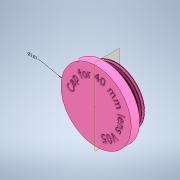
# Autodesk Inventor part: capForSvBonyPlosse-40mmV05
Saved by Autodesk Inventor 2021.1 (Build 251245010, 245A)
## iProperties
Created: 2020-08-18
Part Number: capForSvBonyPlosse-40mmV05
Material: Polycarbonate, Smoke
Document SubType Name: Modeling
Designer: robst
Density: 1.2 g/cm^3
Appearance: Pink
innerDiameter: 0.635 in
heightOfBrake: 0.250 in
majorDiameter: 1.623 in
pitchDiameter: 1.569 in
minorDiameter: 1.524 in
pitch: 0.083 in
crestFlat: 0.017 in
threadsPerInch: 12.000 ul
threadDepth: 0.060 in
Author: robst
Autodesk Inventor part; units mm, degrees
ref_plane "XZ Plane" through (0, 0, 0) normal (0, 1, 0) x (-1, 0, 0)
ref_plane "XY Plane" through (0, 0, 0) normal (0, 0, 1) x (1, 0, 0)
sketch "Sketch1" plane through (0, 0, 0) normal (0, 0, 1) x (1, 0, 0)
  circle A0 centre (0, 0) radius 21.2992
  dimension "d1" = 42.5983
  constraints: 1 centre point
  measures "d1" diameter of A0
extrude "Extrusion1" add sketch "Sketch1" against normal blind 9.525
sketch "Sketch2" plane through (0, 0, 0) normal (0, 0, 1) x (1, 0, 0)
  circle A0 centre (0, 0) radius 26.3436
  dimension "d4" = 52.6872
  constraints: 1 centre point
  measures "d4" diameter of A0
extrude "Extrusion2" add sketch "Sketch2" along normal blind 6.35
sketch "Sketch11" plane through (0, 0, 6.35) normal (0, 0, 1) x (1, 0, 0)
  circle A0 centre (0, 0) radius 19.05 construction
  spline S0 degree 2 poles (-16.2379, 2.4675) (-16.3002, 1.9774) (-16.7363, 1.1904) (-17.1055, 0.9302) knots 0 0 0 1 2 2 2
  spline S1 degree 2 poles (-17.1055, 0.9302) (-17.4706, 0.6695) (-18.4927, 0.4633) (-19.1298, 0.5442) knots 0 0 0 1 2 2 2
  spline S2 degree 2 poles (-19.1298, 0.5442) (-19.7628, 0.6246) (-20.6611, 1.0666) (-20.9693, 1.417) knots 0 0 0 1 2 2 2
  spline S3 degree 2 poles (-20.9693, 1.417) (-21.2699, 1.7622) (-21.5204, 2.6323) (-21.4556, 3.1428) knots 0 0 0 1 2 2 2
  spline S4 degree 2 poles (-21.4556, 3.1428) (-21.4234, 3.396) (-21.2933, 3.8318) (-21.2123, 4.0124) knots 0 0 0 1 2 2 2
  spline S5 degree 2 poles (-21.2123, 4.0124) (-21.1384, 4.169) (-20.9443, 4.4888) (-20.8332, 4.6448) knots 0 0 0 1 2 2 2
  line L0 (-20.8332, 4.6448) -> (-20.0246, 4.5421)
  line L1 (-20.0246, 4.5421) -> (-20.0313, 4.489)
  spline S6 degree 2 poles (-20.0313, 4.489) (-20.1244, 4.4095) (-20.3884, 4.1609) (-20.5241, 3.9748) knots 0 0 0 1 2 2 2
  spline S7 degree 2 poles (-20.5241, 3.9748) (-20.6546, 3.7963) (-20.847, 3.3601) (-20.8843, 3.0661) knots 0 0 0 1 2 2 2
  spline S8 degree 2 poles (-20.8843, 3.0661) (-20.9253, 2.7435) (-20.733, 2.1339) (-20.5073, 1.8853) knots 0 0 0 1 2 2 2
  spline S9 degree 2 poles (-20.5073, 1.8853) (-20.277, 1.6402) (-19.5271, 1.3043) (-19.0411, 1.2425) knots 0 0 0 1 2 2 2
  spline S10 degree 2 poles (-19.0411, 1.2425) (-18.5225, 1.1767) (-17.7435, 1.3308) (-17.4587, 1.5146) knots 0 0 0 1 2 2 2
  spline S11 degree 2 poles (-17.4587, 1.5146) (-17.1826, 1.6953) (-16.8573, 2.2308) (-16.8168, 2.5493) knots 0 0 0 1 2 2 2
  spline S12 degree 2 poles (-16.8168, 2.5493) (-16.78, 2.8393) (-16.8601, 3.3516) (-16.9419, 3.557) knots 0 0 0 1 2 2 2
  spline S13 degree 2 poles (-16.9419, 3.557) (-17.0248, 3.7543) (-17.2105, 4.0559) (-17.2783, 4.1434) knots 0 0 0 1 2 2 2
  line L2 (-17.2783, 4.1434) -> (-17.272, 4.1924)
  line L3 (-17.272, 4.1924) -> (-16.4716, 4.0907)
  spline S14 degree 2 poles (-16.4716, 4.0907) (-16.4153, 3.9134) (-16.3097, 3.6012) (-16.2708, 3.3846) knots 0 0 0 1 2 2 2
  spline S15 degree 2 poles (-16.2708, 3.3846) (-16.2253, 3.1548) (-16.1995, 2.7697) (-16.2379, 2.4675) knots 0 0 0 1 2 2 2
  spline S16 degree 2 poles (-15.5406, 6.7174) (-15.5146, 6.6238) (-15.4158, 6.3044) (-15.402, 6.167) knots 0 0 0 1 2 2 2
  spline S17 degree 2 poles (-15.402, 6.167) (-15.3773, 5.977) (-15.4015, 5.6471) (-15.5039, 5.3777) knots 0 0 0 1 2 2 2
  spline S18 degree 2 poles (-15.5039, 5.3777) (-15.5873, 5.1584) (-15.9035, 4.825) (-16.1106, 4.732) knots 0 0 0 1 2 2 2
  spline S19 degree 2 poles (-16.1106, 4.732) (-16.311, 4.6452) (-16.8078, 4.6359) (-17.0463, 4.7266) knots 0 0 0 1 2 2 2
  spline S20 degree 2 poles (-17.0463, 4.7266) (-17.4157, 4.8671) (-17.8205, 5.3778) (-17.8418, 5.7735) knots 0 0 0 1 2 2 2
  spline S21 degree 2 poles (-17.8418, 5.7735) (-17.8662, 6.1263) (-17.66, 6.9815) (-17.5069, 7.4651) knots 0 0 0 1 2 2 2
  line L4 (-17.5069, 7.4651) -> (-17.6224, 7.509)
  spline S22 degree 2 poles (-17.6224, 7.509) (-17.8301, 7.588) (-18.1362, 7.559) (-18.2532, 7.4714) knots 0 0 0 1 2 2 2
  spline S23 degree 2 poles (-18.2532, 7.4714) (-18.3702, 7.3837) (-18.5423, 7.0704) (-18.6096, 6.8934) knots 0 0 0 1 2 2 2
  spline S24 degree 2 poles (-18.6096, 6.8934) (-18.6886, 6.6856) (-18.7791, 6.077) (-18.7666, 5.7507) knots 0 0 0 1 2 2 2
  line L5 (-18.7666, 5.7507) -> (-18.7797, 5.7161)
  line L6 (-18.7797, 5.7161) -> (-19.3916, 5.9487)
  spline S25 degree 2 poles (-19.3916, 5.9487) (-19.3748, 6.1317) (-19.2547, 6.7951) (-19.1391, 7.0991) knots 0 0 0 1 2 2 2
  spline S26 degree 2 poles (-19.1391, 7.0991) (-18.9986, 7.4685) (-18.6915, 7.9287) (-18.4654, 8.0717) knots 0 0 0 1 2 2 2
  spline S27 degree 2 poles (-18.4654, 8.0717) (-18.2445, 8.2124) (-17.7058, 8.2277) (-17.371, 8.1004) knots 0 0 0 1 2 2 2
  line L7 (-17.371, 8.1004) -> (-14.9353, 7.1743)
  line L8 (-14.9353, 7.1743) -> (-15.1635, 6.574)
  line L9 (-15.1635, 6.574) -> (-15.5406, 6.7174)
  line L10 (-16.0409, 6.9076) -> (-17.0298, 7.2836)
  spline S28 degree 2 poles (-17.0298, 7.2836) (-17.0925, 7.0608) (-17.2743, 6.3857) (-17.2903, 6.1583) knots 0 0 0 1 2 2 2
  spline S29 degree 2 poles (-17.2903, 6.1583) (-17.3079, 5.8919) (-17.1224, 5.4647) (-16.8531, 5.3623) knots 0 0 0 1 2 2 2
  spline S30 degree 2 poles (-16.8531, 5.3623) (-16.5453, 5.2452) (-16.1019, 5.473) (-15.9761, 5.8039) knots 0 0 0 1 2 2 2
  spline S31 degree 2 poles (-15.9761, 5.8039) (-15.8693, 6.0848) (-15.9361, 6.6387) (-16.0409, 6.9076) knots 0 0 0 1 2 2 2
  spline S32 degree 2 poles (-14.4215, 11.7457) (-13.6281, 11.2141) (-13.1975, 9.8303) (-13.5848, 9.2524) knots 0 0 0 1 2 2 2
  spline S33 degree 2 poles (-13.5848, 9.2524) (-13.7429, 9.0164) (-14.0953, 8.7273) (-14.3342, 8.6148) knots 0 0 0 1 2 2 2
  line L11 (-14.3342, 8.6148) -> (-13.0073, 7.7256)
  line L12 (-13.0073, 7.7256) -> (-13.3648, 7.1921)
  line L13 (-13.3648, 7.1921) -> (-17.6977, 10.0958)
  line L14 (-17.6977, 10.0958) -> (-17.3402, 10.6292)
  line L15 (-17.3402, 10.6292) -> (-17.0085, 10.4069)
  spline S34 degree 2 poles (-17.0085, 10.4069) (-17.0568, 10.7268) (-16.9708, 11.3728) (-16.7806, 11.6566) knots 0 0 0 1 2 2 2
  spline S35 degree 2 poles (-16.7806, 11.6566) (-16.4162, 12.2004) (-15.1465, 12.2316) (-14.4215, 11.7457) knots 0 0 0 1 2 2 2
  spline S36 degree 2 poles (-14.7289, 11.1539) (-15.2726, 11.5183) (-16.1026, 11.5739) (-16.3615, 11.1875) knots 0 0 0 1 2 2 2
  spline S37 degree 2 poles (-16.3615, 11.1875) (-16.5128, 10.9618) (-16.5952, 10.4025) (-16.5639, 10.109) knots 0 0 0 1 2 2 2
  line L16 (-16.5639, 10.109) -> (-14.7651, 8.9036)
  spline S38 degree 2 poles (-14.7651, 8.9036) (-14.5261, 9.0457) (-14.2515, 9.2928) (-14.1232, 9.4843) knots 0 0 0 1 2 2 2
  spline S39 degree 2 poles (-14.1232, 9.4843) (-13.8459, 9.8981) (-14.1475, 10.7643) (-14.7289, 11.1539) knots 0 0 0 1 2 2 2
  line L17 (-11.9885, 17.5305) -> (-12.0145, 17.5103)
  spline S40 degree 2 poles (-12.0145, 17.5103) (-12.103, 17.4833) (-12.392, 17.3319) (-12.4927, 17.2536) knots 0 0 0 1 2 2 2
  spline S41 degree 2 poles (-12.4927, 17.2536) (-12.8114, 17.0061) (-12.8623, 16.5079) (-12.5694, 16.1308) knots 0 0 0 1 2 2 2
  line L18 (-12.5694, 16.1308) -> (-12.4911, 16.03)
  line L19 (-12.4911, 16.03) -> (-11.6522, 16.6814)
  line L20 (-11.6522, 16.6814) -> (-11.3265, 16.262)
  line L21 (-11.3265, 16.262) -> (-12.1491, 15.6232)
  line L22 (-12.1491, 15.6232) -> (-10.1366, 13.0319)
  line L23 (-10.1366, 13.0319) -> (-10.6438, 12.638)
  line L24 (-10.6438, 12.638) -> (-12.6563, 15.2293)
  line L25 (-12.6563, 15.2293) -> (-12.9977, 14.9641)
  line L26 (-12.9977, 14.9641) -> (-13.3234, 15.3835)
  line L27 (-13.3234, 15.3835) -> (-12.982, 15.6487)
  line L28 (-12.982, 15.6487) -> (-13.0603, 15.7495)
  spline S42 degree 2 poles (-13.0603, 15.7495) (-13.4795, 16.2892) (-13.3954, 17.2615) (-12.9077, 17.6402) knots 0 0 0 1 2 2 2
  spline S43 degree 2 poles (-12.9077, 17.6402) (-12.7679, 17.7488) (-12.4753, 17.9291) (-12.3496, 17.9955) knots 0 0 0 1 2 2 2
  line L29 (-12.3496, 17.9955) -> (-11.9885, 17.5305)
  spline S44 degree 2 poles (-6.8969, 17.1605) (-6.4569, 16.3035) (-6.8014, 14.9466) (-7.4899, 14.5931) knots 0 0 0 1 2 2 2
  spline S45 degree 2 poles (-7.4899, 14.5931) (-8.1967, 14.2302) (-9.5006, 14.7778) (-9.9255, 15.6055) knots 0 0 0 1 2 2 2
  spline S46 degree 2 poles (-9.9255, 15.6055) (-10.3617, 16.4551) (-10.01, 17.825) (-9.3288, 18.1748) knots 0 0 0 1 2 2 2
  spline S47 degree 2 poles (-9.3288, 18.1748) (-8.6403, 18.5282) (-7.3349, 18.0138) (-6.8969, 17.1605) knots 0 0 0 1 2 2 2
  spline S48 degree 2 poles (-7.4865, 16.8577) (-7.8249, 17.5169) (-8.6337, 17.9115) (-9.0768, 17.684) knots 0 0 0 1 2 2 2
  spline S49 degree 2 poles (-9.0768, 17.684) (-9.52, 17.4565) (-9.6743, 16.5674) (-9.3359, 15.9082) knots 0 0 0 1 2 2 2
  spline S50 degree 2 poles (-9.3359, 15.9082) (-9.0069, 15.2673) (-8.185, 14.8563) (-7.7419, 15.0838) knots 0 0 0 1 2 2 2
  spline S51 degree 2 poles (-7.7419, 15.0838) (-7.3024, 15.3095) (-7.1518, 16.2059) (-7.4865, 16.8577) knots 0 0 0 1 2 2 2
  line L30 (-4.3209, 19.1925) -> (-4.3525, 19.1833)
  spline S52 degree 2 poles (-4.3525, 19.1833) (-4.4294, 19.1823) (-4.5859, 19.1452) (-4.6926, 19.1141) knots 0 0 0 1 2 2 2
  spline S53 degree 2 poles (-4.6926, 19.1141) (-4.9415, 19.0414) (-5.3682, 18.6811) (-5.5272, 18.4032) knots 0 0 0 1 2 2 2
  line L31 (-5.5272, 18.4032) -> (-4.7698, 15.8067)
  line L32 (-4.7698, 15.8067) -> (-5.3863, 15.6269)
  line L33 (-5.3863, 15.6269) -> (-6.4539, 19.2864)
  line L34 (-6.4539, 19.2864) -> (-5.8373, 19.4662)
  line L35 (-5.8373, 19.4662) -> (-5.6783, 18.9209)
  spline S54 degree 2 poles (-5.6783, 18.9209) (-5.43, 19.3192) (-4.9995, 19.7107) (-4.7624, 19.7798) knots 0 0 0 1 2 2 2
  spline S55 degree 2 poles (-4.7624, 19.7798) (-4.6676, 19.8075) (-4.5704, 19.8273) (-4.5077, 19.8327) knots 0 0 0 1 2 2 2
  line L36 (-4.5077, 19.8327) -> (-4.3209, 19.1925)
  line L37 (2.4474, 18.1735) -> (1.8427, 18.1972)
  line L38 (1.8427, 18.1972) -> (1.7743, 16.4531)
  line L39 (1.7743, 16.4531) -> (1.1202, 16.4788)
  line L40 (1.1202, 16.4788) -> (1.1886, 18.2229)
  line L41 (1.1886, 18.2229) -> (-1.0532, 18.3108)
  line L42 (-1.0532, 18.3108) -> (-1.0251, 19.0266)
  line L43 (-1.0251, 19.0266) -> (1.3482, 21.5537)
  line L44 (1.3482, 21.5537) -> (1.9734, 21.5292)
  line L45 (1.9734, 21.5292) -> (1.8642, 18.7443)
  line L46 (1.8642, 18.7443) -> (2.4689, 18.7206)
  line L47 (2.4689, 18.7206) -> (2.4474, 18.1735)
  line L48 (1.2101, 18.77) -> (1.2879, 20.7527)
  line L49 (1.2879, 20.7527) -> (-0.497, 18.837)
  line L50 (-0.497, 18.837) -> (1.2101, 18.77)
  spline S56 degree 2 poles (6.632, 17.9322) (6.2687, 16.6146) (5.1624, 15.5916) (4.3647, 15.8116) knots 0 0 0 1 2 2 2
  spline S57 degree 2 poles (4.3647, 15.8116) (3.5551, 16.0349) (3.144, 17.5019) (3.4997, 18.7917) knots 0 0 0 1 2 2 2
  spline S58 degree 2 poles (3.4997, 18.7917) (3.8653, 20.1172) (4.9694, 21.1323) (5.771, 20.9112) knots 0 0 0 1 2 2 2
  spline S59 degree 2 poles (5.771, 20.9112) (6.5766, 20.689) (6.9844, 19.2101) (6.632, 17.9322) knots 0 0 0 1 2 2 2
  spline S60 degree 2 poles (5.3792, 16.672) (5.5412, 16.8878) (5.8263, 17.612) (5.9653, 18.116) knots 0 0 0 1 2 2 2
  spline S61 degree 2 poles (5.9653, 18.116) (6.1043, 18.62) (6.2296, 19.3841) (6.1993, 19.6614) knots 0 0 0 1 2 2 2
  spline S62 degree 2 poles (6.1993, 19.6614) (6.169, 19.9388) (5.8949, 20.292) (5.6211, 20.3675) knots 0 0 0 1 2 2 2
  spline S63 degree 2 poles (5.6211, 20.3675) (5.3473, 20.443) (4.9229, 20.2825) (4.7486, 20.053) knots 0 0 0 1 2 2 2
  spline S64 degree 2 poles (4.7486, 20.053) (4.5804, 19.8303) (4.2989, 19.088) (4.1664, 18.6078) knots 0 0 0 1 2 2 2
  spline S65 degree 2 poles (4.1664, 18.6078) (4.0242, 18.0919) (3.8972, 17.3839) (3.926, 17.0856) knots 0 0 0 1 2 2 2
  spline S66 degree 2 poles (3.926, 17.0856) (3.9512, 16.8053) (4.2289, 16.4341) (4.5146, 16.3553) knots 0 0 0 1 2 2 2
  spline S67 degree 2 poles (4.5146, 16.3553) (4.7845, 16.2809) (5.2088, 16.4414) (5.3792, 16.672) knots 0 0 0 1 2 2 2
  line L51 (11.9604, 11.5312) -> (13.3681, 13.2304)
  spline S68 degree 2 poles (13.3681, 13.2304) (13.5361, 13.4333) (13.7907, 13.8051) (13.8187, 13.9422) knots 0 0 0 1 2 2 2
  spline S69 degree 2 poles (13.8187, 13.9422) (13.8547, 14.0889) (13.7453, 14.3505) (13.5773, 14.4897) knots 0 0 0 1 2 2 2
  spline S70 degree 2 poles (13.5773, 14.4897) (13.4251, 14.6158) (12.9215, 14.7176) (12.5905, 14.6924) knots 0 0 0 1 2 2 2
  spline S71 degree 2 poles (12.5905, 14.6924) (12.5569, 14.6454) (12.4609, 14.5165) (12.3926, 14.4341) knots 0 0 0 1 2 2 2
  line L52 (12.3926, 14.4341) -> (10.7906, 12.5002)
  line L53 (10.7906, 12.5002) -> (10.2961, 12.9099)
  line L54 (10.2961, 12.9099) -> (11.7037, 14.6091)
  spline S72 degree 2 poles (11.7037, 14.6091) (11.8718, 14.812) (12.1263, 15.1839) (12.1544, 15.321) knots 0 0 0 1 2 2 2
  spline S73 degree 2 poles (12.1544, 15.321) (12.1903, 15.4676) (12.081, 15.7293) (11.9129, 15.8684) knots 0 0 0 1 2 2 2
  spline S74 degree 2 poles (11.9129, 15.8684) (11.7544, 15.9998) (11.2371, 16.0915) (10.9435, 16.0728) knots 0 0 0 1 2 2 2
  line L55 (10.9435, 16.0728) -> (9.1262, 13.8789)
  line L56 (9.1262, 13.8789) -> (8.6317, 14.2886)
  line L57 (8.6317, 14.2886) -> (11.0635, 17.2243)
  line L58 (11.0635, 17.2243) -> (11.5581, 16.8146)
  line L59 (11.5581, 16.8146) -> (11.2902, 16.4912)
  spline S75 degree 2 poles (11.2902, 16.4912) (11.6438, 16.5244) (12.2002, 16.4217) (12.4284, 16.2326) knots 0 0 0 1 2 2 2
  spline S76 degree 2 poles (12.4284, 16.2326) (12.6884, 16.0173) (12.894, 15.446) (12.7754, 15.0898) knots 0 0 0 1 2 2 2
  spline S77 degree 2 poles (12.7754, 15.0898) (13.208, 15.1538) (13.8455, 15.0587) (14.0928, 14.8539) knots 0 0 0 1 2 2 2
  spline S78 degree 2 poles (14.0928, 14.8539) (14.283, 14.6963) (14.4965, 14.3216) (14.5004, 14.0939) knots 0 0 0 1 2 2 2
  spline S79 degree 2 poles (14.5004, 14.0939) (14.5074, 13.8636) (14.3064, 13.3565) (14.057, 13.0553) knots 0 0 0 1 2 2 2
  line L60 (14.057, 13.0553) -> (12.455, 11.1215)
  line L61 (12.455, 11.1215) -> (11.9604, 11.5312)
  line L62 (15.2004, 6.7058) -> (17.1072, 7.8162)
  spline S80 degree 2 poles (17.1072, 7.8162) (17.3348, 7.9488) (17.7019, 8.2102) (17.7755, 8.3293) knots 0 0 0 1 2 2 2
  spline S81 degree 2 poles (17.7755, 8.3293) (17.8597, 8.4545) (17.8472, 8.7378) (17.7374, 8.9264) knots 0 0 0 1 2 2 2
  spline S82 degree 2 poles (17.7374, 8.9264) (17.6379, 9.0971) (17.2002, 9.3662) (16.8808, 9.4565) knots 0 0 0 1 2 2 2
  spline S83 degree 2 poles (16.8808, 9.4565) (16.8331, 9.424) (16.6985, 9.3361) (16.606, 9.2822) knots 0 0 0 1 2 2 2
  line L63 (16.606, 9.2822) -> (14.4359, 8.0185)
  line L64 (14.4359, 8.0185) -> (14.1128, 8.5735)
  line L65 (14.1128, 8.5735) -> (16.0195, 9.6839)
  spline S84 degree 2 poles (16.0195, 9.6839) (16.2472, 9.8165) (16.6143, 10.0778) (16.6878, 10.1969) knots 0 0 0 1 2 2 2
  spline S85 degree 2 poles (16.6878, 10.1969) (16.7721, 10.3222) (16.7596, 10.6055) (16.6498, 10.794) knots 0 0 0 1 2 2 2
  spline S86 degree 2 poles (16.6498, 10.794) (16.5462, 10.9719) (16.0921, 11.2363) (15.8101, 11.3197) knots 0 0 0 1 2 2 2
  line L66 (15.8101, 11.3197) -> (13.3483, 9.8862)
  line L67 (13.3483, 9.8862) -> (13.0251, 10.4411)
  line L68 (13.0251, 10.4411) -> (16.3193, 12.3595)
  line L69 (16.3193, 12.3595) -> (16.6425, 11.8045)
  line L70 (16.6425, 11.8045) -> (16.2796, 11.5932)
  spline S87 degree 2 poles (16.2796, 11.5932) (16.623, 11.5026) (17.11, 11.2145) (17.2591, 10.9583) knots 0 0 0 1 2 2 2
  spline S88 degree 2 poles (17.2591, 10.9583) (17.429, 10.6666) (17.4253, 10.0595) (17.1913, 9.766) knots 0 0 0 1 2 2 2
  spline S89 degree 2 poles (17.1913, 9.766) (17.6194, 9.6771) (18.1852, 9.3682) (18.3468, 9.0907) knots 0 0 0 1 2 2 2
  spline S90 degree 2 poles (18.3468, 9.0907) (18.4711, 8.8772) (18.5425, 8.452) (18.4676, 8.2369) knots 0 0 0 1 2 2 2
  spline S91 degree 2 poles (18.4676, 8.2369) (18.3949, 8.0183) (18.0316, 7.6114) (17.6936, 7.4146) knots 0 0 0 1 2 2 2
  line L71 (17.6936, 7.4146) -> (15.5236, 6.1508)
  line L72 (15.5236, 6.1508) -> (15.2004, 6.7058)
  line L73 (16.3233, 2.4966) -> (16.2139, 3.1294)
  line L74 (16.2139, 3.1294) -> (21.4427, 4.0336)
  line L75 (21.4427, 4.0336) -> (21.5521, 3.4007)
  line L76 (21.5521, 3.4007) -> (16.3233, 2.4966)
  spline S92 degree 2 poles (16.4258, -0.0848) (16.4148, 0.8291) (17.4277, 1.8458) (18.3745, 1.8571) knots 0 0 0 1 2 2 2
  spline S93 degree 2 poles (18.3745, 1.8571) (19.3048, 1.8683) (20.4197, 0.906) (20.4291, 0.1197) knots 0 0 0 1 2 2 2
  spline S94 degree 2 poles (20.4291, 0.1197) (20.4334, -0.2343) (20.2341, -0.7842) (20.0184, -0.9885) knots 0 0 0 1 2 2 2
  spline S95 degree 2 poles (20.0184, -0.9885) (19.8027, -1.197) (19.1755, -1.4227) (18.7186, -1.4282) knots 0 0 0 1 2 2 2
  line L77 (18.7186, -1.4282) -> (18.3687, -1.4324)
  line L78 (18.3687, -1.4324) -> (18.337, 1.2062)
  spline S96 degree 2 poles (18.337, 1.2062) (17.6743, 1.1982) (16.9784, 0.5229) (16.9855, -0.0698) knots 0 0 0 1 2 2 2
  spline S97 degree 2 poles (16.9855, -0.0698) (16.988, -0.2798) (17.0876, -0.6861) (17.1636, -0.8499) knots 0 0 0 1 2 2 2
  spline S98 degree 2 poles (17.1636, -0.8499) (17.2481, -1.0218) (17.395, -1.2588) (17.4618, -1.3363) knots 0 0 0 1 2 2 2
  line L79 (17.4618, -1.3363) -> (17.4622, -1.3733)
  line L80 (17.4622, -1.3733) -> (16.7624, -1.3817)
  spline S99 degree 2 poles (16.7624, -1.3817) (16.7158, -1.2711) (16.5801, -0.9351) (16.5414, -0.8039) knots 0 0 0 1 2 2 2
  spline S100 degree 2 poles (16.5414, -0.8039) (16.4857, -0.6193) (16.4285, -0.3153) (16.4258, -0.0848) knots 0 0 0 1 2 2 2
  spline S101 degree 2 poles (18.851, -0.8008) (19.1103, -0.7895) (19.4877, -0.6779) (19.6141, -0.5735) knots 0 0 0 1 2 2 2
  spline S102 degree 2 poles (19.6141, -0.5735) (19.7568, -0.4606) (19.9049, -0.1089) (19.9018, 0.1505) knots 0 0 0 1 2 2 2
  spline S103 degree 2 poles (19.9018, 0.1505) (19.8987, 0.4057) (19.7421, 0.762) (19.5921, 0.9084) knots 0 0 0 1 2 2 2
  spline S104 degree 2 poles (19.5921, 0.9084) (19.4381, 1.0506) (19.07, 1.1944) (18.8269, 1.2121) knots 0 0 0 1 2 2 2
  line L81 (18.8269, 1.2121) -> (18.851, -0.8008)
  line L82 (15.8012, -5.0184) -> (15.939, -4.3912)
  line L83 (15.939, -4.3912) -> (18.062, -4.8576)
  spline S105 degree 2 poles (18.062, -4.8576) (18.3193, -4.9142) (18.7722, -4.9631) (18.9208, -4.9198) knots 0 0 0 1 2 2 2
  spline S106 degree 2 poles (18.9208, -4.9198) (19.0783, -4.8744) (19.2751, -4.631) (19.3263, -4.3978) knots 0 0 0 1 2 2 2
  spline S107 degree 2 poles (19.3263, -4.3978) (19.3776, -4.1646) (19.2369, -3.6153) (19.088, -3.3339) knots 0 0 0 1 2 2 2
  line L84 (19.088, -3.3339) -> (16.3056, -2.7226)
  line L85 (16.3056, -2.7226) -> (16.4434, -2.0953)
  line L86 (16.4434, -2.0953) -> (20.1667, -2.9133)
  line L87 (20.1667, -2.9133) -> (20.0289, -3.5406)
  line L88 (20.0289, -3.5406) -> (19.6147, -3.4496)
  spline S108 degree 2 poles (19.6147, -3.4496) (19.8062, -3.7867) (19.9523, -4.3878) (19.8852, -4.6934) knots 0 0 0 1 2 2 2
  spline S109 degree 2 poles (19.8852, -4.6934) (19.765, -5.2402) (18.9053, -5.7004) (18.2177, -5.5493) knots 0 0 0 1 2 2 2
  line L89 (18.2177, -5.5493) -> (15.8012, -5.0184)
  spline S110 degree 2 poles (14.9664, -6.7533) (15.1253, -6.405) (15.5875, -5.8873) (15.7829, -5.7366) knots 0 0 0 1 2 2 2
  line L90 (15.7829, -5.7366) -> (16.4384, -6.0354)
  line L91 (16.4384, -6.0354) -> (16.4247, -6.0654)
  spline S111 degree 2 poles (16.4247, -6.0654) (16.3307, -6.113) (16.0961, -6.2504) (15.9406, -6.3831) knots 0 0 0 1 2 2 2
  spline S112 degree 2 poles (15.9406, -6.3831) (15.8028, -6.4967) (15.534, -6.8085) (15.4469, -6.9995) knots 0 0 0 1 2 2 2
  spline S113 degree 2 poles (15.4469, -6.9995) (15.3837, -7.1381) (15.3022, -7.4855) (15.3205, -7.5844) knots 0 0 0 1 2 2 2
  spline S114 degree 2 poles (15.3205, -7.5844) (15.3422, -7.7254) (15.4588, -7.8963) (15.6236, -7.9714) knots 0 0 0 1 2 2 2
  spline S115 degree 2 poles (15.6236, -7.9714) (15.8296, -8.0653) (16.1456, -7.9379) (16.3483, -7.6819) knots 0 0 0 1 2 2 2
  spline S116 degree 2 poles (16.3483, -7.6819) (16.4257, -7.5815) (16.6646, -7.2561) (16.7758, -7.1213) knots 0 0 0 1 2 2 2
  spline S117 degree 2 poles (16.7758, -7.1213) (17.073, -6.7772) (17.7164, -6.6362) (18.0572, -6.7916) knots 0 0 0 1 2 2 2
  spline S118 degree 2 poles (18.0572, -6.7916) (18.5292, -7.0068) (18.7945, -7.9828) (18.5281, -8.5672) knots 0 0 0 1 2 2 2
  spline S119 degree 2 poles (18.5281, -8.5672) (18.3966, -8.8556) (17.9879, -9.375) (17.7887, -9.524) knots 0 0 0 1 2 2 2
  line L92 (17.7887, -9.524) -> (17.1632, -9.2388)
  line L93 (17.1632, -9.2388) -> (17.1768, -9.2089)
  spline S120 degree 2 poles (17.1768, -9.2089) (17.4591, -9.0661) (17.9145, -8.6132) (18.0425, -8.3322) knots 0 0 0 1 2 2 2
  spline S121 degree 2 poles (18.0425, -8.3322) (18.174, -8.0438) (18.1116, -7.5357) (17.8681, -7.4247) knots 0 0 0 1 2 2 2
  spline S122 degree 2 poles (17.8681, -7.4247) (17.6471, -7.324) (17.326, -7.4626) (17.139, -7.6941) knots 0 0 0 1 2 2 2
  spline S123 degree 2 poles (17.139, -7.6941) (17.0473, -7.8061) (16.833, -8.0975) (16.7115, -8.2547) knots 0 0 0 1 2 2 2
  spline S124 degree 2 poles (16.7115, -8.2547) (16.4399, -8.5924) (15.8166, -8.7787) (15.4308, -8.6028) knots 0 0 0 1 2 2 2
  spline S125 degree 2 poles (15.4308, -8.6028) (15.206, -8.5004) (14.8892, -8.1433) (14.8217, -7.9044) knots 0 0 0 1 2 2 2
  spline S126 degree 2 poles (14.8217, -7.9044) (14.7518, -7.6508) (14.8042, -7.1092) (14.9664, -6.7533) knots 0 0 0 1 2 2 2
  line L94 (13.8627, -16.6824) -> (11.4874, -11.8631)
  line L95 (11.4874, -11.8631) -> (12.0004, -11.3457)
  line L96 (12.0004, -11.3457) -> (16.8396, -13.6802)
  line L97 (16.8396, -13.6802) -> (16.3294, -14.1947)
  line L98 (16.3294, -14.1947) -> (12.3418, -12.2234)
  line L99 (12.3418, -12.2234) -> (14.3468, -16.1942)
  line L100 (14.3468, -16.1942) -> (13.8627, -16.6824)
  spline S127 degree 2 poles (8.5255, -17.1132) (7.8142, -15.9462) (7.8263, -14.4394) (8.5329, -14.0088) knots 0 0 0 1 2 2 2
  spline S128 degree 2 poles (8.5329, -14.0088) (9.25, -13.5718) (10.6006, -14.2769) (11.2969, -15.4194) knots 0 0 0 1 2 2 2
  spline S129 degree 2 poles (11.2969, -15.4194) (12.0124, -16.5935) (11.996, -18.0932) (11.2859, -18.526) knots 0 0 0 1 2 2 2
  spline S130 degree 2 poles (11.2859, -18.526) (10.5723, -18.9609) (9.2153, -18.2452) (8.5255, -17.1132) knots 0 0 0 1 2 2 2
  spline S131 degree 2 poles (8.4652, -15.3373) (8.5115, -15.6032) (8.8439, -16.3069) (9.116, -16.7533) knots 0 0 0 1 2 2 2
  spline S132 degree 2 poles (9.116, -16.7533) (9.3881, -17.1998) (9.8591, -17.8143) (10.0819, -17.9822) knots 0 0 0 1 2 2 2
  spline S133 degree 2 poles (10.0819, -17.9822) (10.3048, -18.1501) (10.7498, -18.1922) (10.9924, -18.0444) knots 0 0 0 1 2 2 2
  spline S134 degree 2 poles (10.9924, -18.0444) (11.235, -17.8965) (11.4086, -17.4774) (11.3607, -17.1932) knots 0 0 0 1 2 2 2
  spline S135 degree 2 poles (11.3607, -17.1932) (11.3136, -16.9181) (10.9655, -16.2046) (10.7063, -15.7793) knots 0 0 0 1 2 2 2
  spline S136 degree 2 poles (10.7063, -15.7793) (10.4278, -15.3223) (9.9988, -14.7449) (9.7617, -14.5616) knots 0 0 0 1 2 2 2
  spline S137 degree 2 poles (9.7617, -14.5616) (9.5402, -14.388) (9.0795, -14.3361) (8.8264, -14.4904) knots 0 0 0 1 2 2 2
  spline S138 degree 2 poles (8.8264, -14.4904) (8.5874, -14.6361) (8.4138, -15.0553) (8.4652, -15.3373) knots 0 0 0 1 2 2 2
  spline S139 degree 2 poles (4.1909, -17.7) (4.0765, -17.3519) (4.1041, -16.6842) (4.2355, -16.3984) knots 0 0 0 1 2 2 2
  spline S140 degree 2 poles (4.2355, -16.3984) (4.3669, -16.1125) (4.8896, -15.6591) (5.2651, -15.5358) knots 0 0 0 1 2 2 2
  spline S141 degree 2 poles (5.2651, -15.5358) (5.6092, -15.4227) (6.332, -15.3542) (6.6183, -15.3944) knots 0 0 0 1 2 2 2
  line L101 (6.6183, -15.3944) -> (6.8432, -16.0789)
  line L102 (6.8432, -16.0789) -> (6.7962, -16.0943)
  spline S142 degree 2 poles (6.7962, -16.0943) (6.7039, -16.0639) (6.38, -16.0144) (6.1912, -16.0071) knots 0 0 0 1 2 2 2
  spline S143 degree 2 poles (6.1912, -16.0071) (5.9778, -16.0036) (5.6366, -16.0333) (5.4371, -16.0989) knots 0 0 0 1 2 2 2
  spline S144 degree 2 poles (5.4371, -16.0989) (5.2415, -16.1631) (4.9202, -16.4247) (4.8373, -16.6209) knots 0 0 0 1 2 2 2
  spline S145 degree 2 poles (4.8373, -16.6209) (4.7636, -16.8055) (4.7644, -17.2299) (4.8492, -17.488) knots 0 0 0 1 2 2 2
  spline S146 degree 2 poles (4.8492, -17.488) (4.934, -17.7461) (5.1828, -18.0284) (5.3517, -18.0942) knots 0 0 0 1 2 2 2
  spline S147 degree 2 poles (5.3517, -18.0942) (5.5285, -18.1705) (5.9686, -18.1385) (6.215, -18.0576) knots 0 0 0 1 2 2 2
  spline S148 degree 2 poles (6.215, -18.0576) (6.481, -17.9702) (6.982, -17.7146) (7.1307, -17.6267) knots 0 0 0 1 2 2 2
  line L103 (7.1307, -17.6267) -> (7.948, -20.114)
  line L104 (7.948, -20.114) -> (5.3003, -20.984)
  line L105 (5.3003, -20.984) -> (5.114, -20.4169)
  line L106 (5.114, -20.4169) -> (7.1399, -19.7513)
  line L107 (7.1399, -19.7513) -> (6.7171, -18.4646)
  spline S149 degree 2 poles (6.7171, -18.4646) (6.6049, -18.5188) (6.3819, -18.605) (6.288, -18.6359) knots 0 0 0 1 2 2 2
  spline S150 degree 2 poles (6.288, -18.6359) (5.9165, -18.758) (5.3643, -18.8051) (5.0705, -18.7023) knots 0 0 0 1 2 2 2
  spline S151 degree 2 poles (5.0705, -18.7023) (4.7729, -18.6007) (4.3348, -18.138) (4.1909, -17.7) knots 0 0 0 1 2 2 2
  dimension "d57" = 38.1
  constraints: 1 centre point, 1 coincident, 1 other
  measures "d57" diameter of A0
extrude "Extrusion4" cut sketch "Sketch11" against normal blind 1.27
sketch "Sketch12" plane through (0, 0, -9.525) normal (0, 0, -1) x (-1, 0, 0)
  circle A0 centre (0, 0) radius 15.24
  dimension "d60" = 30.48
  constraints: 1 centre point, 1 coincident
  measures "d60" diameter of A0
extrude "Extrusion5" cut sketch "Sketch12" against normal blind 12.7
sketch "Sketch15" plane through (0, 0, 0) normal (1, 0, 0) x (0, 1, 0)
  line L0 (20.0863, -9.525) -> (21.195, -10.1651) construction
  line L1 (21.195, -10.5259) -> (20.0863, -11.166)
  line L2 (20.0863, -11.5267) -> (21.195, -12.1668)
  line L3 (21.195, -12.5276) -> (20.0863, -13.1677) construction
  arc A0 (21.195, -10.5259) -> (21.195, -10.1651) centre (21.0909, -10.3455) ccw
  arc A1 (20.0863, -11.166) -> (20.0863, -11.5267) centre (20.1905, -11.3464) ccw
  arc A2 (21.195, -12.5276) -> (21.195, -12.1668) centre (21.0909, -12.3472) ccw
  line L4 (20.0863, -9.525) -> (27.2471, -9.525) construction
  line L5 (0, -15.8013) -> (0, 2.6335) construction
  line L6 (-21.2992, -9.525) -> (21.2992, -9.525) construction
  line L7 (21.2992, -10.3455) -> (21.2992, -12.3472)
  point P0 (0, 0)
  dimension "d89" = 60
  dimension "d93" = 30
  dimension "d94" = 19.9822
  dimension "d95" = 21.2992
  dimension "d96" = 0
  dimension "d97" = 0.2083
  constraints: 12 end point, 8 point on circle, 6 tangent, 3 centre point, 3 equal length, 2 equal radius, 1 horizontal
  measures "d89" angle of L2 L1
  measures "d93" angle of L0 L4
  measures "d94" distance edge to line of A1 L5
  measures "d96" distance between parallel lines of L4 L6
  measures "d97" radius of A1
coil "Coil4" sketch "Sketch15" operation cut axis through (0, 0, -10) along (0, 0, 1) pitch 2.1167 turns 6 hand right
equation "\"d1\" = a1MajorDiameterAvg"
equation "\"d2\" = threadPostLength"
equation "\"d4\" = handleDiameter"
equation "\"d5\" = handleLength"
equation "\"d94\" = 0.5 * a1MinorDiameterAvg"
equation "\"d95\" = 0.5 * a1MajorDiameterAvg"
equation "\"d97\" = a1RootRadiusAvg"
equation "\"d98\" = pitch"
equation "\"handleDiameter\" = 52.68722"
equation "\"brakeHandle\" = 30deg"
equation "\"innerDiameter\" = 16.129"
equation "\"heightOfBrake\" = 6.35"
equation "\"majorDiameter\" = 41.22928"
equation "\"pitchDiameter\" = 39.85514"
equation "\"minorDiameter\" = 38.7096"
equation "\"crestFlat\" = 0.4318"
equation "\"threadsPerInch\" = 12"
equation "\"threadDepth\" = 1.52146"
equation "\"totalLength\" = 15.875"
equation "\"handleLength\" = 6.35"
equation "\"threadPostLength\" = totalLength - handleLength"
equation "\"threadLength\" = threadPostLength + 2 * pitch"
equation "\"brakeStopLength\" = 12.7"
equation "\"a1MajorDiameterAvg\" = 42.59834"
equation "\"a1MinorDiameterAvg\" = 39.96436"
equation "\"a1RootRadiusAvg\" = 0.20828"
equation "\"pitch\" = 2.116667"
body "Solid1"
